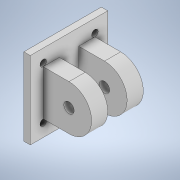
# Autodesk Inventor part: Undercarriage load
Saved by Autodesk Inventor 2020 (Build 240168000, 168)
## iProperties
Created: 2021-01-30
Part Number: Undercarriage load
Material: Generic
Document SubType Name: Modeling
Designer: magda
Density: 1 g/cm^3
Appearance: Default
Author: magda
Autodesk Inventor part; units mm, degrees
ref_plane "YZ Plane" through (0, 0, 0) normal (1, 0, 0) x (0, 1, 0)
ref_plane "XZ Plane" through (0, 0, 0) normal (0, 1, 0) x (-1, 0, 0)
ref_plane "XY Plane" through (0, 0, 0) normal (0, 0, 1) x (1, 0, 0)
sketch "Sketch1" plane through (0, 0, 0) normal (1, 0, 0) x (0, 1, 0)
  line L0 (22.5602, 53.0087) -> (-53.6398, 53.0087)
  line L1 (-53.6398, 53.0087) -> (-53.6398, -23.1913)
  line L2 (-53.6398, -23.1913) -> (22.5602, -23.1913)
  line L3 (22.5602, -23.1913) -> (22.5602, 53.0087)
  point P0 (0, 0)
  dimension "d0" = 76.2
  dimension "d1" = 76.2
  constraints: 8 end point, 2 parallel, 1 horizontal, 1 perpendicular
  measures "d0" distance of L2.end L0.start
  measures "d1" distance of L1.end L2.end
extrude "Extrusion1" add sketch "Sketch1" along normal blind 6.35
sketch "Sketch2" plane through (6.35, 0, 0) normal (1, 0, 0) x (0, 0, -1)
  line L0 (23.1913, 22.5602) -> (-53.0087, 22.5602) projected
  line L1 (-53.0087, 22.5602) -> (-53.0087, -53.6398) projected
  line L2 (23.1913, -53.6398) -> (23.1913, 22.5602) projected
  line L3 (-53.0087, -53.6398) -> (23.1913, -53.6398) projected
  point P0 (0, 0)
  point P1 (-40.3087, 9.8602)
  point P2 (10.4913, 9.8602)
  point P3 (-40.3087, -40.9398)
  point P4 (10.4913, -40.9398)
  dimension "d4" = 12.7
  dimension "d5" = 12.7
  dimension "d6" = 12.7
  dimension "d7" = 12.7
  dimension "d8" = 12.7
  dimension "d9" = 12.7
  dimension "d10" = 12.7
  dimension "d11" = 12.7
  measures "d4" distance from line of L0 point (-40.309, 9.86)
  measures "d5" distance from line of L1 point (-40.309, 9.86)
  measures "d6" distance from line of L2 point (10.491, 9.86)
  measures "d7" distance from line of L0 point (10.491, 9.86)
  measures "d8" distance from line of L2 point (10.491, -40.94)
  measures "d9" distance from line of L3 point (10.491, -40.94)
  measures "d10" distance from line of L1 point (-40.309, -40.94)
  measures "d11" distance from line of L3 point (-40.309, -40.94)
hole "Hole1" at (6.35, 9.8602, 40.3087) at (6.35, 9.8602, -10.4913) at (6.35, -40.9398, 40.3087) at (6.35, -40.9398, -10.4913) direction (-1, 0, 0) diameter 6.35 end through all
sketch "Sketch3" plane through (0, -53.6398, 53.0087) normal (0, 0, 1) x (1, 0, 0)
  line L0 (6.35, 76.2) -> (6.35, 0) projected
  line L1 (6.35, 60.325) -> (31.75, 60.325)
  line L2 (31.75, 60.325) -> (31.75, 15.875)
  line L3 (31.75, 15.875) -> (6.35, 15.875)
  line L4 (6.35, 15.875) -> (6.35, 60.325)
  line L5 (0, 76.2) -> (6.35, 76.2) projected
  arc A0 (31.75, 15.875) -> (31.75, 60.325) centre (31.75, 38.1) ccw
  circle A1 centre (31.75, 38.1) radius 5.08
  point P0 (0, 53.6398)
  point P1 (6.35, 15.875)
  dimension "d19" = 25.4
  dimension "d20" = 44.45
  dimension "d21" = 15.875
  dimension "d22" = 10.16
  constraints: 8 end point, 2 centre point, 2 parallel, 2 point on circle, 1 coincident, 1 horizontal, 1 midpoint, 1 perpendicular, 1 point on line
  measures "d19" distance of L2.end L3.end
  measures "d20" distance of L1.end L2.end
  measures "d21" distance between parallel lines of L5 L1
  measures "d22" diameter of A1
extrude "Extrusion2" add sketch "Sketch3" against normal blind 76.2 contours L1 L2 A1 L3 L0 | A0 L2 A1
sketch "Sketch4" plane through (6.35, 6.6852, 53.0087) normal (0, 1, 0) x (1, 0, 0)
  line L0 (25.4, 0) -> (0, 0) projected
  line L1 (0, 0) -> (74.1036, 0)
  line L2 (74.1036, 0) -> (74.1036, 12.7)
  line L3 (74.1036, 12.7) -> (0, 12.7)
  line L4 (0, 12.7) -> (0, 0)
  line L5 (-6.35, 76.2) -> (0, 76.2) projected
  line L6 (0, 76.2) -> (74.1036, 76.2)
  line L7 (74.1036, 76.2) -> (74.1036, 63.5)
  line L8 (74.1036, 63.5) -> (0, 63.5)
  line L9 (0, 63.5) -> (0, 76.2)
  line L10 (0, 28.575) -> (74.1036, 28.575)
  line L11 (74.1036, 28.575) -> (74.1036, 47.625)
  line L12 (74.1036, 47.625) -> (0, 47.625)
  line L13 (0, 47.625) -> (0, 28.575)
  point P0 (-6.35, 53.0087)
  dimension "d25" = 12.7
  dimension "d26" = 12.7
  dimension "d27" = 19.05
  dimension "d28" = 15.875
  constraints: 24 end point, 6 parallel, 3 horizontal, 3 perpendicular, 1 point on line
  measures "d25" distance between parallel lines of L6 L8
  measures "d26" distance between parallel lines of L1 L3
  measures "d27" distance between parallel lines of L12 L10
  measures "d28" distance between parallel lines of L3 L10
extrude "Extrusion3" cut sketch "Sketch4" against normal blind 76.2
body "Solid1"
